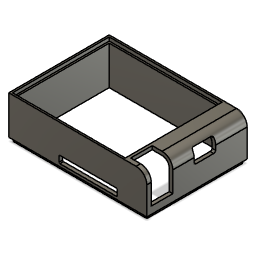
Tapa2_Intermedia Final (Autodesk Fusion 360 design; units mm, degrees)
Autodesk Fusion 360 part; units mm, degrees
sketch "Boceto1" plane through (0, 0, 0) normal (0, 0, 1) x (1, 0, 0)
  line L0 (0, 0) -> (77, 0)
  line L1 (77, 0) -> (77, 23.5)
  line L2 (77, 23.5) -> (0, 23.5)
  line L3 (0, 23.5) -> (0, 0)
  dimension "d1" = 77
  dimension "d2" = 23.5
  constraint horizontal L0
  constraint vertical L1
  constraint horizontal L2
  constraint vertical L3
  constraint coincident L0.start L3.end
  measures "d1" distance of L0.start L0.end
  measures "d2" distance of L0.end L1.end
extrude "Extruir1" add sketch "Boceto1" along normal blind 56
shell "Vaciado1" thickness 2 removed faces 1 at (25.6667, 0, 18.6667)
sketch "Boceto2" plane through (0, 23.5, 0) normal (0, 1, 0) x (-1, 0, 0)
  line L0 (-77, 0) -> (0, 0)
  line L1 (0, 0) -> (0, 56)
  line L2 (0, 56) -> (-77, 56)
  line L3 (-77, 56) -> (-77, 0)
  line L4 (-1, 1) -> (-64, 1)
  line L5 (-64, 1) -> (-64, 55)
  line L6 (-64, 55) -> (-1, 55)
  line L7 (-1, 55) -> (-1, 1)
  dimension "d6" = 1
  dimension "d7" = 1
  dimension "d8" = 1
  dimension "d9" = 63
  constraint horizontal L4
  constraint vertical L5
  constraint horizontal L6
  constraint vertical L7
  measures "d6" distance of L0 L4
  measures "d7" distance of L1 L7
  measures "d8" distance of L2 L6
  measures "d9" distance of L5 L7
extrude "Extruir2" cut sketch "Boceto2" against normal blind 2 contours L4 L5 L6 L7
sketch "Boceto3" plane through (0, 0, 0) normal (0, -1, 0) x (1, 0, 0)
  line L0 (2, 2) -> (2, 54)
  line L1 (2, 54) -> (75, 54)
  line L2 (75, 54) -> (75, 2)
  line L3 (75, 2) -> (2, 2)
  line L4 (0, 0) -> (77, 0)
  line L5 (77, 0) -> (77, 56)
  line L6 (77, 56) -> (0, 56)
  line L7 (0, 56) -> (0, 0)
  line L8 (1.2, 1.2) -> (75.8, 1.2)
  line L9 (75.8, 1.2) -> (75.8, 54.8)
  line L10 (75.8, 54.8) -> (1.2, 54.8)
  line L11 (1.2, 54.8) -> (1.2, 1.2)
  dimension "d12" = -1.2
extrude "Extruir3" cut sketch "Boceto3" against normal blind 2 contours L4 L5 L6 L7
sketch "Boceto4" plane through (0, 23.5, 0) normal (0, 1, 0) x (-1, 0, 0)
  line L0 (-64, 1) -> (-64, 55)
  line L1 (-64, 55) -> (-1, 55)
  line L2 (-1, 55) -> (-1, 1)
  line L3 (-1, 1) -> (-64, 1)
  line L4 (-77, 0) -> (0, 0)
  line L5 (0, 0) -> (0, 56)
  line L6 (0, 56) -> (-77, 56)
  line L7 (-77, 56) -> (-77, 0)
  line L8 (-77, 53.5) -> (-65.5, 53.5)
  line L9 (-65.5, 53.5) -> (-65.5, 41.5)
  line L10 (-65.5, 41.5) -> (-77, 41.5)
  line L11 (-77, 41.5) -> (-77, 53.5)
  dimension "d15" = 2.5
  dimension "d16" = 11.5
  dimension "d17" = 12
  constraint horizontal L8
  constraint vertical L9
  constraint horizontal L10
  constraint vertical L11
  constraint coincident L7 L8.start
  measures "d15" distance of L6 L8
  measures "d16" distance of L9 L11
  measures "d17" distance of L8.end L9.end
extrude "Extruir4" cut sketch "Boceto4" against normal blind 17.5 contours L7 L8 L9 L10 L11
sketch "Boceto5" plane through (77, 0, 0) normal (1, 0, 0) x (0, 0, -1)
  line L0 (-41.5, 23.5) -> (-41.5, 6)
  line L1 (-41.5, 6) -> (-53.5, 6)
  line L2 (-53.5, 6) -> (-53.5, 23.5)
  line L3 (-53.5, 23.5) -> (-56, 23.5)
  line L4 (-56, 23.5) -> (-56, 2)
  line L5 (-56, 2) -> (0, 2)
  line L6 (0, 2) -> (0, 23.5)
  line L7 (0, 23.5) -> (-41.5, 23.5)
  line L8 (-29.6, 21.5) -> (-17.6, 21.5)
  line L9 (-17.6, 21.5) -> (-17.6, 14)
  line L10 (-17.6, 14) -> (-29.6, 14)
  line L11 (-29.6, 14) -> (-29.6, 21.5)
  dimension "d20" = 7.5
  dimension "d21" = 12
  dimension "d22" = 2
  dimension "d23" = 17.6
  constraint horizontal L8
  constraint vertical L9
  constraint horizontal L10
  constraint vertical L11
  measures "d20" distance of L8.end L9.end
  measures "d21" distance of L8.start L8.end
  measures "d22" distance of L7 L8
  measures "d23" distance of L6 L9
extrude "Extruir5" cut sketch "Boceto5" against normal blind 2 contours L8 L9 L10 L11
fillet "Empalme1" radius 1 4 edges at (76, 21.5, 17.6) (76, 14, 17.6) (76, 14, 29.6) (76, 21.5, 29.6)
fillet "Empalme3" radius 6 2 edges at (77, 23.5, 20.75) (77, 23.5, 54.75)
fillet "Empalme3" radius 4 3 edges at (75, 21.5, 35.05) (75, 21.5, 10.3) (75, 21.5, 53.75)
sketch "Boceto6" plane through (0, 0, 56) normal (0, 0, 1) x (1, 0, 0)
  arc A0 (77, 17.5) -> (71, 23.5) centre (71, 17.5) ccw
  line L0 (71, 23.5) -> (0, 23.5)
  line L1 (0, 23.5) -> (0, 2)
  line L2 (0, 2) -> (77, 2)
  line L3 (77, 2) -> (77, 17.5)
  line L4 (28, 7.5) -> (60.5, 7.5)
  line L5 (60.5, 7.5) -> (60.5, 3.5)
  line L6 (60.5, 3.5) -> (28, 3.5)
  line L7 (28, 3.5) -> (28, 7.5)
  dimension "d40" = 1.5
  dimension "d41" = 16.5
  dimension "d42" = 4
  dimension "d43" = 32.5
  constraint horizontal L4
  constraint vertical L5
  constraint horizontal L6
  constraint vertical L7
  measures "d40" distance of L2 L6
  measures "d41" distance of L3 L5
  measures "d42" distance of L4.end L5.end
  measures "d43" distance of L4.start L4.end
extrude "Extruir6" cut sketch "Boceto6" against normal blind 2 contours L4 L5 L6 L7
fillet "Empalme4" radius 0.5 4 edges at (60.5, 7.5, 55) (60.5, 3.5, 55) (28, 3.5, 55) (28, 7.5, 55)
